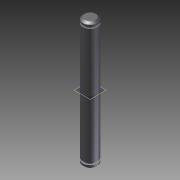
# Autodesk Inventor part: TU-009
Saved by Autodesk Inventor 2011 (Build 150229000, 229)
## iProperties
Shininess: 64.0
Angle Display Precision: 2
Document Length Units: 11269
Document Angle Units: 11279
Document Time Units: 11290
Document Mass Units: 11286
Document Length Units Precision: 3
Document Angle Units Precision: 2
Compacted: True
Created: 2002-07-24
Part Number: TU-009
Document SubType Name: Modeling
Designer: PN
Description: Long Pin
Density: 8.08 g/cm^3
Mass: 27.8886 g
Surface Area: 19.0317 cm^2
Volume: 3.45156 cm^3
Material: Stainless Steel
Density: 0.0
Volumn: 0.0
Area: 0.0
PropertySet Name: Model Information
Control State: 0
Master: False
Checked Out: False
LENGTH: 1.000 in
Author: PN
Autodesk Inventor part; units mm, degrees
ref_plane "YZ Plane" through (0, 0, 0) normal (1, 0, 0) x (0, 1, 0)
ref_plane "XZ Plane" through (0, 0, 0) normal (0, 1, 0) x (-1, 0, 0)
ref_plane "XY Plane" through (0, 0, 0) normal (0, 0, 1) x (1, 0, 0)
sketch "Sketch1" plane through (0, 0, 0) normal (0, 0, 1) x (1, 0, 0)
  line L0 (0, 70) -> (3, 70)
  line L1 (3, 70) -> (4, 69)
  line L2 (4, 69) -> (4, 68)
  line L3 (4, 68) -> (3, 68)
  line L4 (3, 68) -> (3, 67)
  line L5 (3, 67) -> (4, 67)
  line L6 (4, 67) -> (4, 3)
  line L7 (4, 3) -> (3, 3)
  line L8 (3, 3) -> (3, 2)
  line L9 (3, 2) -> (4, 2)
  line L10 (4, 2) -> (4, 1)
  line L11 (4, 1) -> (3, 0)
  line L12 (0, 70) -> (0, 0)
  line L13 (0, 0) -> (3, 0)
  dimension "d4" = 65
  dimension "d5" = 1
  dimension "d6" = 66
  dimension "d7" = 2
  dimension "d19" = 8
  dimension "d20" = 45
  dimension "d23" = 1
  dimension "d24" = 1
  constraints: 28 end point, 5 perpendicular, 3 collinear, 2 equal length, 1 coincident, 1 horizontal, 1 parallel
  measures "d4" distance between parallel lines of L3 L7
  measures "d5" distance between parallel lines of L3 L5
  measures "d6" distance between parallel lines of L3 L9
  measures "d7" distance between parallel lines of L3 L0
  measures "d19" diameter of L10 L12
  measures "d20" angle of L13 L11
  measures "d23" distance from line of L11.end L10
  measures "d24" distance between parallel lines of L4 L6
revolve "Revolution1" add sketch "Sketch1" angle 360 about axis through (0, 70, 0) along (0, -1, 0)
ref_plane "Work Plane1" through (0, 35, 0) normal (0, -1, 0) x (1, 0, 0)
equation "\"LENGTH\" = 25.4"
body "Solid1"
